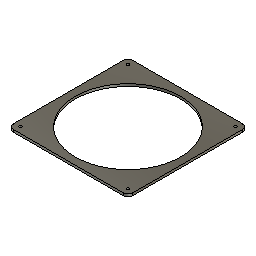
WateringSystemHIL_PCBHolder v1 (Autodesk Fusion 360 design; units mm, degrees)
Autodesk Fusion 360 part; units mm, degrees
sketch "Sketch1" plane through (0, 0, 0) normal (0, 0, 1) x (1, 0, 0)
  line L0 (4, 0) -> (96, 0)
  line L1 (100, 4) -> (100, 96)
  line L2 (96, 100) -> (4, 100)
  line L3 (0, 96) -> (0, 4)
  arc A0 (0, 4) -> (4, 0) centre (4, 4) ccw
  arc A1 (4, 100) -> (0, 96) centre (4, 96) ccw
  arc A2 (100, 96) -> (96, 100) centre (96, 96) ccw
  arc A3 (96, 0) -> (100, 4) centre (96, 4) ccw
  circle A4 centre (50, 49.9614) radius 44
  circle A5 centre (5, 95) radius 1.05
  circle A6 centre (95, 95) radius 1.05
  circle A7 centre (95, 5) radius 1.05
  circle A8 centre (5, 5) radius 1.05
  point P0 (100, 0)
  point P1 (0, 100)
  dimension "d1" = 100
  dimension "d2" = 100
  dimension "d3" = 4
  dimension "d4" = 4
  dimension "d5" = 4
  dimension "d6" = 4
  dimension "d7" = 88
  dimension "d8" = 2.1
  dimension "d9" = 2.1
  dimension "d10" = 2.1
  dimension "d11" = 2.1
  constraint horizontal L0
  constraint vertical L1
  constraint horizontal L2
  constraint vertical L3
  constraint coincident origin L0
  constraint coincident origin L3
  constraint tangent L0 A0
  constraint tangent L3 A0
  constraint coincident P1 L2
  constraint coincident P1 L3
  constraint tangent L2 A1
  constraint tangent L3 A1
  constraint tangent L1 A2
  constraint tangent L2 A2
  constraint coincident P0 L0
  constraint coincident P0 L1
  constraint tangent L0 A3
  constraint tangent L1 A3
  measures "d1" distance of origin P0
  measures "d2" distance of origin P1
  measures "d3" radius of A0
  measures "d4" radius of A1
  measures "d5" radius of A2
  measures "d6" radius of A3
  measures "d7" diameter of A4
  measures "d8" diameter of A5
  measures "d9" diameter of A6
  measures "d10" diameter of A7
  measures "d11" diameter of A8
extrude "Extrude1" add sketch "Sketch1" along normal blind 2
